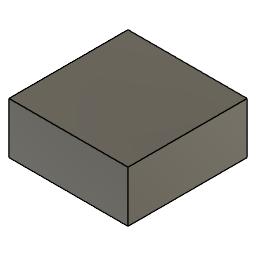
popup-1.0 (Autodesk Fusion 360 design; units mm, degrees)
part number: 2026-05-20-10-52-14-662
part number: 2026-05-20-10-55-48-825
Autodesk Fusion 360 part; units mm, degrees
sketch "base" plane through (0, 0, 0) normal (0, 0, 1) x (1, 0, 0) in component "base"
  line L0 (50, 50) -> (-50, 50)
  line L1 (-50, 50) -> (-50, -50)
  line L2 (-50, -50) -> (50, -50)
  line L3 (50, -50) -> (50, 50)
  line L4 (50, 50) -> (-50, -50) construction
  line L5 (-50, 50) -> (50, -50) construction
  dimension "d1" = 100
  dimension "d2" = 100
  constraint horizontal L0
  constraint perpendicular L0 L1
  constraint parallel L0 L2
  constraint parallel L1 L3
  constraint coincident L4 origin
  constraint coincident L5 origin
  measures "d1" distance of L1.end L2.end
  measures "d2" distance of L0.end L1.end
extrude "Extrude1" add sketch "base" along normal blind 3 in component "base"
sketch "legs" plane through (0, 0, 0) normal (0, 0, -1) x (1, 0, 0) in component "base"
  line L0 (50, -50) -> (50, 50)
  line L1 (50, 50) -> (-50, 50)
  line L2 (-50, 50) -> (-50, -50)
  line L3 (-50, -50) -> (50, -50)
  line L4 (47.5, 47.5) -> (-47.5, 47.5)
  line L5 (-47.5, 47.5) -> (-47.5, -47.5)
  line L6 (-47.5, -47.5) -> (47.5, -47.5)
  line L7 (47.5, -47.5) -> (47.5, 47.5)
  line L8 (47.5, 47.5) -> (-47.5, -47.5) construction
  line L9 (-47.5, 47.5) -> (47.5, -47.5) construction
  line L10 (-50, -50) -> (50, -50)
  line L11 (50, -50) -> (50, 50)
  line L12 (50, 50) -> (-50, 50)
  line L13 (-50, 50) -> (-50, -50)
  dimension "d5" = 95
  dimension "d6" = 95
  dimension "d7" = 2.5
  constraint horizontal L4
  constraint perpendicular L4 L5
  constraint parallel L4 L6
  constraint parallel L5 L7
  constraint coincident L8 origin
  constraint coincident L9 origin
  measures "d5" distance of L5.end L6.end
  measures "d6" distance of L4.end L5.end
extrude "Extrude2" add sketch "legs" along normal blind 40 in component "base"
component "base" placed x (1, 0, 0) y (0, 1, 0) z (0, 0, 1) at (0, 0, 0)
named bodies: "base"
